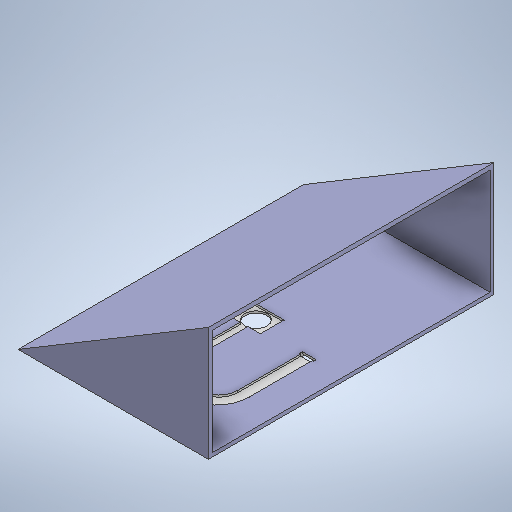
# Autodesk Inventor part: PitchedRoof
Saved by Autodesk Inventor 2026.2 (Build 302298010, 298A)
## iProperties
Created: 2026-03-19
Part Number: PitchedRoof
Material: Ogólny
Document SubType Name: Modeling
Designer: Patryk
Density: 1 g/cm^3
Appearance: Domyślna
Author: Patryk
Autodesk Inventor part; units mm, degrees
ref_plane "YZ Plane" through (0, 0, 0) normal (1, 0, 0) x (0, 1, 0)
ref_plane "XZ Plane" through (0, 0, 0) normal (0, 1, 0) x (-1, 0, 0)
ref_plane "XY Plane" through (0, 0, 0) normal (0, 0, 1) x (1, 0, 0)
sketch "Szkic1" plane through (0, 0, 0) normal (0, 0, 1) x (1, 0, 0)
  line L0 (0, 0) -> (-200, 0)
  line L1 (0, 0) -> (0, 120)
  line L2 (0, 120) -> (-200, 0)
  dimension "d0" = 200
  dimension "d1" = 120
  constraints: 6 end point, 1 horizontal, 1 vertical
  measures "d0" distance of L0.start L0.end
  measures "d1" distance of L0.start L1.end
extrude "Wyciągnięcie proste1" add sketch "Szkic1" along normal mid plane 300
shell "Skorupa1" thickness 4 removed faces 1 at (0, 40, -50)
sketch "Szkic2" plane through (-185.5587, 4, -146) normal (0, 1, 0) x (1, 0, 0)
  line L0 (68.5587, -133.5) -> (102.5587, -133.5)
  line L1 (102.5587, -133.5) -> (102.5587, -158.5)
  line L2 (102.5587, -158.5) -> (68.5587, -158.5)
  line L3 (68.5587, -158.5) -> (68.5587, -133.5)
  line L4 (185.5587, 4) -> (-14.4413, 4) projected
  line L5 (185.5587, 4) -> (185.5587, -296) projected
  circle A0 centre (85.5587, -146) radius 11.5
  point P0 (185.5587, -146)
  dimension "d5" = 34
  dimension "d6" = 25
  dimension "d7" = 137.5
  dimension "d8" = 83
  dimension "d9" = 23
  dimension "d10" = 100
  dimension "d11" = 150
  constraints: 8 end point, 2 parallel, 1 centre point, 1 horizontal, 1 perpendicular
  measures "d5" distance of L1.end L2.end
  measures "d6" distance of L0.end L1.end
  measures "d7" distance between parallel lines of L4 L0
  measures "d8" distance between parallel lines of L5 L1
  measures "d9" diameter of A0
  measures "d10" distance from line of L5 A0.centre
  measures "d11" distance from line of A0.centre L4
extrude "Wyciągnięcie proste2" cut sketch "Szkic2" against normal through all contours A0
extrude "Wyciągnięcie proste3" cut sketch "Szkic2" against normal blind 2
sketch "Szkic3" plane through (-200, 0, 150) normal (0, -1, 0) x (1, 0, 0)
  circle A0 centre (100, -150) radius 11.5 projected
  line L0 (200, -300) -> (200, 0) projected
  line L1 (0, 0) -> (200, 0) projected
  line L2 (0, 0) -> (0, -300) projected
  line L3 (200, -300) -> (0, -300) projected
  line L4 (155.5, -159.75) -> (170, -159.75)
  line L5 (170, -159.75) -> (170, -140.25)
  line L6 (170, -140.25) -> (155.5, -140.25)
  line L7 (155.5, -140.25) -> (155.5, -159.75)
  line L8 (155.5, -159.75) -> (170, -140.25) construction
  line L9 (170, -159.75) -> (155.5, -140.25) construction
  line L10 (170, -143.25) -> (155.5, -143.25)
  point P0 (200, -150)
  point P1 (162.75, -150)
  dimension "d16" = 14.5
  dimension "d17" = 19.5
  dimension "d18" = 140.25
  dimension "d19" = 30
  dimension "d20" = 3
  constraints: 14 end point, 2 horizontal, 2 midpoint, 2 parallel, 2 point on line, 1 perpendicular
  measures "d16" distance of L6.end L5.end
  measures "d17" distance of L5.end L4.end
  measures "d18" distance between parallel lines of L3 L4
  measures "d19" distance between parallel lines of L0 L5
  measures "d20" distance between parallel lines of L10 L6
extrude "Wyciągnięcie proste4" cut sketch "Szkic3" against normal blind 2 contours L7 L10 L5 L4
extrude "Wyciągnięcie proste5" cut sketch "Szkic3" against normal blind 4 contours L7 L6 L5 L10
sketch "Szkic4" plane through (-185.5587, 4, -146) normal (0, 1, 0) x (1, 0, 0)
  line L0 (141.0587, -152.75) -> (155.5587, -152.75) projected
  line L1 (155.5587, -152.75) -> (155.5587, -155.75) projected
  line L2 (155.5587, -155.75) -> (141.0587, -155.75) projected
  line L3 (141.0587, -155.75) -> (141.0587, -152.75) projected
  line L4 (102.5587, -133.5) -> (102.5587, -158.5) projected
  line L5 (102.5587, -158.5) -> (68.5587, -158.5) projected
  line L6 (68.5587, -158.5) -> (68.5587, -133.5) projected
  line L7 (68.5587, -133.5) -> (102.5587, -133.5) projected
  line L8 (185.5587, 0) -> (185.5587, -292) projected
  line L9 (185.5587, 0) -> (0, 0) projected
  line L10 (0, -292) -> (0, 0) projected
  line L11 (0, -292) -> (185.5587, -292) projected
  line L12 (81.5587, -158.5) -> (89.5587, -158.5)
  line L13 (89.5587, -158.5) -> (89.5587, -222)
  line L14 (89.5587, -292) -> (81.5587, -292)
  line L15 (81.5587, -222) -> (81.5587, -158.5)
  line L16 (141.0587, -155.75) -> (155.5587, -155.75)
  line L17 (155.5587, -292) -> (141.0587, -292)
  line L18 (142.3087, -155.75) -> (154.3087, -155.75)
  line L19 (154.3087, -155.75) -> (154.3087, -222)
  line L20 (154.3087, -292) -> (142.3087, -292)
  line L21 (142.3087, -222) -> (142.3087, -155.75)
  line L22 (109.3319, -242) -> (124.3319, -242)
  line L23 (124.3319, -242) -> (124.3319, -292)
  line L24 (124.3319, -292) -> (109.3319, -292)
  line L25 (109.3319, -292) -> (109.3319, -242)
  line L26 (109.3319, -242) -> (109.5587, -242)
  line L27 (124.3319, -242) -> (122.3087, -242)
  line L28 (109.3319, -257) -> (116.5587, -257)
  line L29 (124.3319, -257) -> (119.3087, -257)
  arc A0 (89.5587, -222) -> (109.5587, -242) centre (109.5587, -222) ccw
  arc A1 (81.5587, -222) -> (116.5587, -257) centre (116.5587, -222) ccw
  arc A2 (122.3087, -242) -> (142.3087, -222) centre (122.3087, -222) ccw
  arc A3 (119.3087, -257) -> (154.3087, -222) centre (119.3087, -222) ccw
  line L30 (124.3319, -257) -> (124.3319, -256.6377)
  point P0 (185.5587, -146)
  point P1 (124.3319, -267)
  point P2 (116.8319, -292)
  point P3 (142.3087, -242)
  point P4 (89.5587, -257)
  point P5 (142.3087, -257)
  point P6 (109.3319, -256.2458)
  dimension "d25" = 96
  dimension "d26" = 8
  dimension "d28" = 31.25
  dimension "d29" = 12
  dimension "d33" = 15
  dimension "d34" = 61.2269
  dimension "d36" = 50
  dimension "d37" = 30
  dimension "d38" = 30
  dimension "d39" = 44.5
  dimension "d40" = 35
  dimension "d41" = 20
  dimension "d42" = 35
  dimension "d43" = 20
  dimension "d44" = 35
  constraints: 38 end point, 22 point on line, 9 point on circle, 8 tangent, 7 parallel, 5 perpendicular, 4 centre point, 4 horizontal, 2 midpoint
  measures "d25" distance between parallel lines of L8 L13
  measures "d26" distance between parallel lines of L13 L15
  measures "d28" distance between parallel lines of L8 L19
  measures "d29" distance between parallel lines of L19 L21
  measures "d33" distance of L22.start L22.end
  measures "d34" distance from line of L8 point (124.332, -267)
  measures "d36" distance from line of point (116.832, -292) L22
  measures "d37" distance from line of L16.end L8
  measures "d38" distance from line of L17.start L8
  measures "d39" distance from line of L17.end L8
  measures "d40" distance between parallel lines of L11 L28
  measures "d41" radius of A0
  measures "d42" radius of A1
  measures "d43" radius of A2
  measures "d44" radius of A3
extrude "Wyciągnięcie proste6" cut sketch "Szkic4" against normal blind 2 contours L2 L19 A3 L23 L22 A2 L21 | L22 L23 A3 L29 L11 L25 L28 A1 | L23 L29 A3 | L25 A1 L15 L5 L13 A0 | A1 L28 L25
